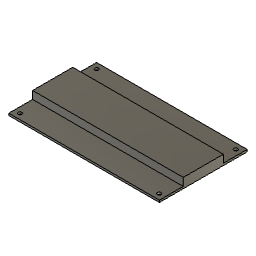
load_cell_holder v10 (Autodesk Fusion 360 design; units mm, degrees)
Autodesk Fusion 360 part; units mm, degrees
note: some values were not read from the file. Set by a fixed rule: which face or edge a step refers to.
sketch "Sketch1" plane through (0, 0, 0) normal (0, 0, 1) x (1, 0, 0)
  line L0 (0, 0) -> (100, 0)
  line L1 (100, 0) -> (100, 60)
  line L2 (100, 60) -> (0, 60)
  line L3 (0, 60) -> (0, 0)
  dimension "d1" = 100
  dimension "d2" = 60
  constraint horizontal L0
  constraint vertical L1
  constraint horizontal L2
  constraint vertical L3
  constraint coincident L0.start L3.end
  measures "d1" distance of L0.start L0.end
  measures "d2" distance of L0.start L2.end
extrude "Extrude1" add sketch "Sketch1" along normal blind 15 makes body 1
sketch "Sketch2" plane through (0, 0, 15) normal (0, 0, 1) x (-1, 0, 0)
  line L0 (0, -60) -> (0, 0)
  line L1 (0, 0) -> (-100, 0)
  line L2 (-100, 0) -> (-100, -60)
  line L3 (-100, -60) -> (0, -60)
  line L4 (-10, -20) -> (-20, -20)
  line L5 (-20, -20) -> (-20, -40)
  line L6 (-20, -40) -> (-10, -40)
  line L7 (-10, -40) -> (-10, -20)
  constraint horizontal L4
  constraint vertical L5
  constraint horizontal L6
  constraint vertical L7
extrude "Extrude2" add sketch "Sketch2" along normal blind 60 contours L4 L5 L6 L7 bodies 1
sketch "Sketch3" plane through (0, 0, 75) normal (0, 0, 1) x (-1, 0, 0)
  line L0 (-10, -40) -> (-10, -20)
  line L1 (-10, -20) -> (-20, -20)
  line L2 (-20, -20) -> (-20, -40)
  line L3 (-20, -40) -> (-10, -40)
  circle A0 centre (-15, -33) radius 1.5
  circle A1 centre (-15, -27) radius 1.5
  dimension "d11" = 3
  dimension "d12" = 3
  measures "d11" diameter of A0
  measures "d12" diameter of A1
extrude "Extrude3" cut sketch "Sketch3" against normal blind 10 contours A0 | A1 bodies 1
copy_body "Body->Comp1" bodies 1 removing the originals makes body 2 in component "Holder"
sketch "Sketch4" plane through (0, 0, 0) normal (0, 0, 1) x (1, 0, 0)
  circle A0 centre (0, 0) radius 20
  dimension "d15" = 40
  constraint coincident A0.centre origin
  measures "d15" diameter of A0
sketch "Sketch5" plane through (0, 0, 10) normal (0, 0, 1) x (-1, 0, 0)
  circle A0 centre (0, 0) radius 20
  circle A1 centre (3, 0) radius 1.5
  circle A2 centre (-3, 0) radius 1.5
  dimension "d20" = 3
  dimension "d21" = 3
  dimension "d22" = 3
  dimension "d23" = 3
  measures "d20" distance of A0.centre A2.centre
  measures "d21" distance of A0.centre A1.centre
  measures "d22" diameter of A1
  measures "d23" diameter of A2
sketch "Sketch6" plane through (0, 0, 0) normal (0, 0, -1) x (1, 0, 0)
  circle A0 centre (3, 0) radius 1.5
  circle A1 centre (-3, 0) radius 1.5
  circle A2 centre (0, 0) radius 20
  circle A3 centre (-3, 0) radius 3.5
  circle A4 centre (3, 0) radius 3.5
  dimension "d26" = 7
  dimension "d27" = 7
  constraint concentric A1 A3
  constraint concentric A0 A4
  measures "d26" diameter of A3
  measures "d27" diameter of A4
sketch "Sketch7" plane through (0, 0, 20) normal (0, 0, 1) x (-1, 0, 0)
  circle A0 centre (3, 0) radius 1.5
  circle A1 centre (-3, 0) radius 1.5
  circle A2 centre (-3, 0) radius 3
  circle A3 centre (3, 0) radius 3
  circle A4 centre (0, 0) radius 20
  dimension "d38" = 6
  dimension "d39" = 6
  constraint concentric A1 A2
  constraint concentric A0 A3
  measures "d38" diameter of A2
  measures "d39" diameter of A3
sketch "Sketch8" plane through (0, 0, 0) normal (0, 0, 1) x (1, 0, 0)
  circle A0 centre (0, 0) radius 30
  dimension "d44" = 60
  constraint coincident A0.centre origin
  measures "d44" diameter of A0
extrude "Extrude9" add sketch "Sketch8" along normal blind 10 separate body makes body 3
sketch "Sketch9" plane through (0, 0, 10) normal (0, 0, 1) x (-1, 0, 0)
  circle A0 centre (0, 0) radius 30
  circle A1 centre (3, 0) radius 1.5
  circle A2 centre (-3, 0) radius 1.5
  dimension "d48" = 3
  dimension "d49" = 3
  measures "d48" diameter of A1
  measures "d49" diameter of A2
extrude "Extrude10" cut sketch "Sketch9" against normal blind 10 contours A1 | A2 bodies 3
sketch "Sketch10" plane through (0, 0, 0) normal (0, 0, -1) x (1, 0, 0)
  circle A0 centre (-3, 0) radius 1.5
  circle A1 centre (3, 0) radius 1.5
  circle A2 centre (0, 0) radius 30
  line L0 (7, 4) -> (-7, 4)
  line L1 (-7, 4) -> (-7, -4)
  line L2 (-7, -4) -> (7, -4)
  line L3 (7, -4) -> (7, 4)
  line L4 (7, 4) -> (-7, -4) construction
  line L5 (-7, 4) -> (7, -4) construction
  constraint horizontal L0
  constraint perpendicular L0 L1
  constraint parallel L0 L2
  constraint parallel L1 L3
  constraint coincident L4 A2.centre
  constraint coincident L5 A2.centre
  constraint coincident A2.centre origin
extrude "Extrude11" add sketch "Sketch10" along normal blind 5 contours L0 L1 L2 L3 bodies 3
sketch "Sketch11" plane through (0, 0, 10) normal (0, 0, 1) x (-1, 0, 0)
  circle A0 centre (3, 0) radius 1.5
  circle A1 centre (-3, 0) radius 1.5
  circle A2 centre (0, 0) radius 30
  circle A3 centre (-3, 0) radius 3
  circle A4 centre (3, 0) radius 3
  dimension "d54" = 6
  dimension "d55" = 6
  constraint concentric A1 A3
  constraint concentric A0 A4
  measures "d54" diameter of A3
  measures "d55" diameter of A4
extrude "Extrude12" cut sketch "Sketch11" against normal blind 3.5 contours A3 | A4 bodies 3
fillet "Fillet4" radius 1 4 edges at (0, -4, -5) (-7, 0, -5) (7, 0, -5) (0, 4, -5) on bodies 3
fillet "Fillet5" radius 1 1 edges at (-27.9698, -10.8485, 10) on bodies 3
fillet "Fillet6" radius 2 4 edges at (0, -4, 0) (0, 4, 0) (-7, 0, 0) (7, 0, 0) on bodies 3
copy_body "Body->Comp3" bodies 3 removing the originals makes body 4 in component "Cap"
sketch "Sketch13" plane through (0, 0, 0) normal (0, 0, 1) x (1, 0, 0)
  circle A0 centre (-27, 0) radius 5
  dimension "d66" = 27
  dimension "d67" = 10
  measures "d66" distance of origin A0.centre
  measures "d67" diameter of A0
combine "Combine1" [no effect]
sketch "Sketch14" plane through (0, 0, 0) normal (0, 0, 1) x (1, 0, 0)
sketch "Sketch15" plane through (0, 0, 0) normal (1, 0, 0) x (0, 1, 0)
  line L0 (31, 170) -> (-31, 170)
  constraint horizontal L0
sketch "Sketch16" plane through (0, 0, 0) normal (0, 0, 1) x (1, 0, 0)
  line L0 (0, 30) -> (0, -31)
sketch "Sketch17" plane through (0, 0, 0) normal (0, 1, 0) x (1, 0, 0)
  line L0 (-30, -170) -> (-30, -130)
  line L1 (-30, -130) -> (-15, -130)
  constraint vertical L0
  constraint perpendicular L0 L1
sketch "Sketch18" plane through (0, 0, 0) normal (0, 0, 1) x (1, 0, 0)
sketch "Sketch19" plane through (0, 0, 0) normal (1, 0, 0) x (0, 1, 0)
sketch "Sketch20" plane through (0, 0, 0) normal (1, 0, 0) x (0, 1, 0)
sketch "Sketch21" plane through (0, 0, 0) normal (0, 1, 0) x (1, 0, 0)
  line L0 (-22, -130) -> (-22, -166)
  constraint vertical L0
sketch "Sketch22" plane through (0, 0, 0) normal (0, 0, 1) x (1, 0, 0)
  line L0 (-2, 30) -> (10, 30)
  constraint horizontal L0
sketch "Sketch23" plane through (0, 0, 0) normal (0, 1, 0) x (1, 0, 0)
sketch "Sketch24" plane through (0, 0, 0) normal (0, 1, 0) x (1, 0, 0)
  arc A0 (56, -167) -> (5, -90) centre (-23.7184, -164.4109) ccw
sketch "Sketch25" plane through (0, 0, 0) normal (0, 1, 0) x (1, 0, 0)
sketch "Sketch26" plane through (0, 0, 0) normal (0, 1, 0) x (1, 0, 0)
sketch "Sketch27" plane through (0, 0, 0) normal (0, 0, 1) x (1, 0, 0)
  circle A0 centre (0, 0) radius 15
  dimension "d78" = 30
  constraint coincident A0.centre origin
  measures "d78" diameter of A0
ref_plane "WorkPlane1" through (0, 0, 150) normal (0, 0, 1) x (1, 0, 0)
sketch "Sketch28" plane through (0, 0, 150) normal (0, 0, 1) x (1, 0, 0)
  circle A0 centre (0, 0) radius 60
  dimension "d80" = 120
  constraint coincident A0.centre origin
  measures "d80" diameter of A0
sketch "Sketch29" plane through (0, 0, 0) normal (0, 0, -1) x (1, 0, 0)
  circle A0 centre (0, 0) radius 15
  circle A1 centre (0, 0) radius 13.5
  dimension "d82" = 27
  constraint coincident A0.centre A1.centre
  measures "d82" diameter of A1
sketch "Sketch30" plane through (0, 0, 0) normal (0, 1, 0) x (1, 0, 0)
move_face "OffsetFaces1" offset -30 1 faces at (14.9626, 38.1653, 75) on bodies 2 in component "Holder"
extrude "Extrude1'" cut 2 faces at (15.1761, 33.4442, 65) (14.5056, 27.0745, 65) along direction (0, 0, -1) blind 40 on bodies 2 bodies 2 in component "Holder"
sketch "Sketch31" plane through (0, 0, 0) normal (0, 0, 1) x (1, 0, 0)
  line L0 (0, 0) -> (120, 0)
  line L1 (120, 0) -> (120, 70)
  line L2 (120, 70) -> (0, 70)
  line L3 (0, 70) -> (0, 0)
  dimension "d88" = 120
  dimension "d89" = 70
  constraint horizontal L0
  constraint vertical L1
  constraint horizontal L2
  constraint vertical L3
  constraint coincident L0.start L3.end
  measures "d88" distance of L0.start L0.end
  measures "d89" distance of L0.start L2.end
extrude "Extrude15" add sketch "Sketch31" along normal blind 1.6 separate body makes body 5
sketch "Sketch32" plane through (0, 0, 1.6) normal (0, 0, 1) x (-1, 0, 0)
  line L0 (0, -70) -> (0, 0)
  line L1 (0, 0) -> (-120, 0)
  line L2 (-120, 0) -> (-120, -70)
  line L3 (-120, -70) -> (0, -70)
  line L4 (0, -19) -> (-120, -19)
  line L5 (-120, -19) -> (-120, -51)
  line L6 (-120, -51) -> (0, -51)
  constraint horizontal L4
  constraint vertical L5
  constraint horizontal L6
  constraint coincident L2 L5.end
extrude "Extrude16" add sketch "Sketch32" along normal blind 6.2 contours L0 L2 L4 L5 L6 bodies 5
sketch "Sketch33" plane through (0, 0, 0) normal (0, 0, -1) x (1, 0, 0)
  line L0 (0, 0) -> (0, -70)
  line L1 (0, -70) -> (120, -70)
  line L2 (120, -70) -> (120, 0)
  line L3 (120, 0) -> (0, 0)
  line L4 (0, 0) -> (3.5, 0)
  line L5 (0, 0) -> (0, -3.5)
  line L6 (3.5, 0) -> (0, 0)
  line L7 (0, 0) -> (0, -3.5)
  circle A0 centre (4.6218, -4.4958) radius 1.5
  circle A1 centre (115.3782, -4.4958) radius 1.5
  circle A2 centre (4.6218, -65.5042) radius 1.5
  circle A3 centre (115.3782, -65.5042) radius 1.5
  dimension "d96" = 3.5
  dimension "d97" = 3.5
  dimension "d98" = 3
  constraint coincident L0.start L3.end
  constraint perpendicular L0 L4
  constraint perpendicular L3 L5
  constraint horizontal L6
  constraint vertical L7
  measures "d96" distance of L0.start L4.end
  measures "d97" distance of L0.start L5.end
  measures "d98" diameter of A0
extrude "Extrude17" cut sketch "Sketch33" against normal blind 10 contours A0 | A1 | A2 | A3 bodies 5
component "Holder" placed x (1, 0, 0) y (0, 1, 0) z (0, 0, 1) at (0, 0, 0)
component "Cap" placed x (1, 0, 0) y (0, 1, 0) z (0, 0, 1) at (0, 0, 0)
